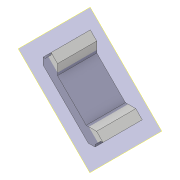
# Autodesk Inventor part: 20_Cube_Insert_Mirror_Holder_30x30Mirror_v2
Saved by Autodesk Inventor 2019 (Build 230136000, 136)
## iProperties
Created: 2019-07-22
Part Number: 20_Cube_Insert_Mirror_Holder_30x30Mirror_v2
Material: Generic
Document SubType Name: Modeling
Designer: diederichbenedict
Density: 1 g/cm^3
Appearance: Default
Author: diederichbenedict
Autodesk Inventor part; units mm, degrees
ref_plane "YZ Plane" through (0, 0, 0) normal (1, 0, 0) x (0, 1, 0)
ref_plane "XZ Plane" through (0, 0, 0) normal (0, 1, 0) x (-1, 0, 0)
ref_plane "XY Plane" through (0, 0, 0) normal (0, 0, 1) x (1, 0, 0)
sketch "Sketch1" plane through (0, 0, 0) normal (0, 0, 1) x (1, 0, 0)
  line L0 (-16.9, 21.4) -> (-16.9, 16.9) construction
  arc A0 (-22.9, 19.9) -> (-19.9, 22.9) centre (-19.9, 19.9) ccw construction
  line L1 (-16.9, 16.9) -> (16.9, 16.9) construction
  line L2 (16.9, 16.9) -> (16.9, -16.9) construction
  line L3 (16.9, -16.9) -> (-16.9, -16.9) construction
  line L4 (-16.9, -16.9) -> (-16.9, 16.9) construction
  arc A1 (22.9, -19.9) -> (19.9, -22.9) centre (19.9, -19.9) ccw construction
  line L5 (22.9, 19.9) -> (22.9, -19.9) construction
  arc A2 (19.9, 22.9) -> (22.9, 19.9) centre (19.9, 19.9) ccw construction
  line L6 (-19.9, 22.9) -> (19.9, 22.9) construction
  arc A3 (-22.9, 19.9) -> (-19.9, 22.9) centre (-19.9, 19.9) ccw construction
  line L7 (-22.9, -19.9) -> (-22.9, 19.9) construction
  arc A4 (-19.9, -22.9) -> (-22.9, -19.9) centre (-19.9, -19.9) ccw construction
  line L8 (19.9, -22.9) -> (-19.9, -22.9) construction
  line L9 (-21.4, 16.9) -> (-16.9, 16.9) construction
  line L10 (-16.9, -16.9) -> (-21.4, -16.9) construction
  line L11 (-16.9, -16.9) -> (-16.9, -21.4) construction
  line L12 (16.9, -21.4) -> (16.9, -16.9) construction
  line L13 (21.4, -16.9) -> (16.9, -16.9) construction
  line L14 (16.9, 16.9) -> (21.4, 16.9) construction
  line L15 (16.9, 16.9) -> (16.9, 21.4) construction
  line L16 (-16.8009, 21.2415) -> (21.2415, -16.8009)
  line L17 (21.2415, -16.8009) -> (16.8009, -21.2415)
  line L18 (16.8009, -21.2415) -> (-21.2415, 16.8009)
  line L19 (-21.2415, 16.8009) -> (-16.8009, 21.2415)
  line L20 (-16.8009, 21.2415) -> (16.8009, -21.2415) construction
  line L21 (21.2415, -16.8009) -> (-21.2415, 16.8009) construction
  line L22 (-16.8009, 21.2415) -> (36.9991, 21.2415) construction
  line L23 (-21.2415, 16.8009) -> (-22.9, 16.8009)
  line L24 (16.8009, -21.2415) -> (16.8009, -22.9)
  line L25 (16.8009, -22.9) -> (-22.9, 16.8009)
  line L26 (-16.8009, 21.2415) -> (-16.8009, 22.9)
  line L27 (21.2415, -16.8009) -> (22.9, -16.8009)
  line L28 (22.9, -16.8009) -> (-16.8009, 22.9)
  line L29 (-22.9, 16.8009) -> (-22.9, 11.5863)
  line L30 (16.8009, -22.9) -> (11.5863, -22.9)
  line L31 (-22.9, 11.5863) -> (11.5863, -22.9)
  point P0 (0, 0)
  dimension "d0" = 53.8
  dimension "d1" = 45
  dimension "d2" = 6.28
  dimension "d5" = 8
  constraints: 32 end point, 6 point on line, 4 parallel, 4 perpendicular, 2 midpoint, 1 equal length, 1 horizontal
  measures "d0" distance of L16.start L16.end
  measures "d1" angle of L16 L22
  measures "d2" distance of L16.end L17.end
  measures "d5" distance from line of L31 point (0, 0)
extrude "Extrusion1" add sketch "Sketch1" along normal blind 30
ref_plane "Work Plane1" through (16.9, -16.9, -8) normal (-0.7071, -0.7071, 0) x (0, 0, 1)
sketch "Sketch7" plane through (0, 0, 30) normal (0, 0, 1) x (1, 0, 0)
  line L0 (21.2415, -16.8009) -> (22.9, -16.8009) projected
  line L1 (22.9, -16.8009) -> (-16.8009, 22.9) projected
  line L2 (-16.8009, 22.9) -> (-16.8009, 21.2415) projected
  line L3 (-16.8009, 21.2415) -> (-21.2415, 16.8009) projected
  line L4 (-21.2415, 16.8009) -> (-22.9, 16.8009) projected
  line L5 (-22.9, 16.8009) -> (-22.9, 11.5863) projected
  line L6 (-22.9, 11.5863) -> (11.5863, -22.9) projected
  line L7 (11.5863, -22.9) -> (16.8009, -22.9) projected
  line L8 (16.8009, -22.9) -> (16.8009, -21.2415) projected
  line L9 (16.8009, -21.2415) -> (21.2415, -16.8009) projected
  line L10 (3.0496, 3.0496) -> (-5.6569, -5.6569)
  line L11 (-22.9, 11.5863) -> (11.5863, -22.9) projected
  line L12 (17.9785, -3.9418) -> (10.0409, -11.8794)
  line L13 (10.0409, -11.8794) -> (-11.8794, 10.0409)
  line L14 (-11.8794, 10.0409) -> (-3.9418, 17.9785)
  line L15 (-3.9418, 17.9785) -> (17.9785, -3.9418)
  line L16 (17.9785, -3.9418) -> (-11.8794, 10.0409) construction
  line L17 (10.0409, -11.8794) -> (-3.9418, 17.9785) construction
  line L18 (-11.8794, 10.0409) -> (-11.8794, 17.9785)
  line L19 (22.9, -16.8009) -> (-16.8009, 22.9) projected
  line L20 (10.0409, -11.8794) -> (17.9785, -11.8794)
  point P0 (0, 0)
  dimension "d28" = 31
  dimension "d29" = 1.3
  constraints: 18 end point, 4 midpoint, 2 parallel, 2 perpendicular, 2 point on line, 1 vertical
  measures "d28" distance of L12.end L13.end
  measures "d29" distance from line of L13 point (0, 0)
extrude "Extrusion7" cut sketch "Sketch7" against normal through all contours L20 L12 L1 | L12 L13 L10 L1 | L1 L14 L15 L12 | L10 L13 L14 L1 | L14 L18 L1
equation "\"d3\" = MirrorThickness1"
equation "\"MirrorThickness1\" = 30"
body "Solid1"
